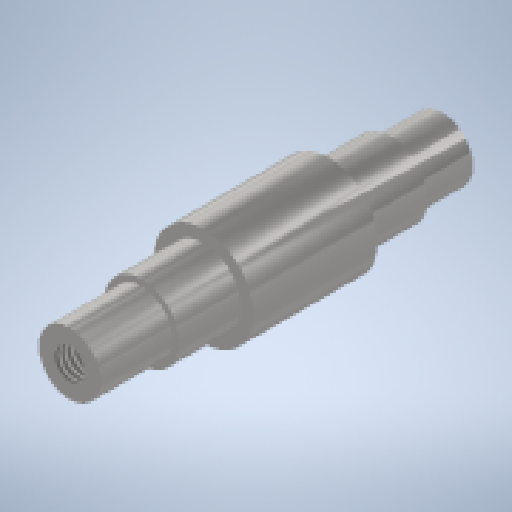
# Autodesk Inventor part: TorquimeterShaft
Saved by Autodesk Inventor 2025 (Build 290162000, 162)
## iProperties
Created: 2024-04-04
Part Number: TorquimeterShaft
Material: Stainless Steel, Austenitic
Document SubType Name: Modeling
Designer: Vinicius
Density: 8 g/cm^3
Appearance: Semi-Polished
Mass: 12.0637 g
Surface Area: 8.54513 cm^2
Volume: 1.50796 cm^3
Author: Vinicius
Autodesk Inventor part; units mm, degrees
ref_plane "YZ Plane" through (0, 0, 0) normal (1, 0, 0) x (0, 1, 0)
ref_plane "XZ Plane" through (0, 0, 0) normal (0, 1, 0) x (-1, 0, 0)
ref_plane "XY Plane" through (0, 0, 0) normal (0, 0, 1) x (1, 0, 0)
sketch "Sketch1" plane through (0, 0, 0) normal (0, 1, 0) x (-1, 0, 0)
  line L0 (0, 0) -> (2.5, 0)
  line L1 (2.5, 0) -> (2.5, -26.2)
  line L2 (2.5, -26.2) -> (0, -26.2)
  line L3 (0, -26.2) -> (0, 0)
  line L4 (2.5, -5.8) -> (3, -5.8)
  line L5 (3, -5.8) -> (3, -11)
  line L6 (3, -11) -> (4, -11)
  line L7 (4, -11) -> (4, -21)
  line L8 (4, -21) -> (3, -21)
  line L9 (3, -21) -> (3, -26.2)
  line L10 (3, -26.2) -> (2.5, -26.2)
  dimension "d0" = 5
  dimension "d10" = 6
  dimension "d11" = 5.8
  dimension "d12" = 8
  dimension "d13" = 5.2
  dimension "d14" = 5.2
  dimension "d15" = 10
  constraints: 23 end point, 7 perpendicular, 3 point on line, 2 parallel, 1 horizontal, 1 vertical alignment
  measures "d0" diameter of L1 L3
  measures "d10" diameter of L5 L3
  measures "d11" distance from line of L0.end L4
  measures "d12" diameter of L7 L3
  measures "d13" distance of L4.end L5.end
  measures "d14" distance of L8.end L9.end
  measures "d15" distance of L6.end L7.end
revolve "Revolution1" add sketch "Sketch1" angle 360 about axis through (0, 0, -26.2) along (0, 0, 1)
sketch "Sketch2" plane through (0, 0, 0) normal (0, 0, 1) x (1, 0, 0)
  point P0 (0, 0)
  point P1 (0, 0)
  constraints: 1 coincident
hole "Hole1" at (0, 0, 0) direction (0, 0, -1) diameter 2.459 depth 7.8 tip angle 118 thread size "M3x0.5" class "6H" standard "ISO Metric profile"
sketch "Sketch3" plane through (0, 0, -26.2) normal (0, 0, -1) x (-1, 0, 0)
  circle A0 centre (0, 0) radius 1.2295 projected
  point P0 (0, 0)
  constraints: 1 coincident
hole "Hole2" at (0, 0, -26.2) direction (0, 0, 1) diameter 3 depth 3.1 tip angle 118
equation "\"d14\" = d13"
body "Solid1"
